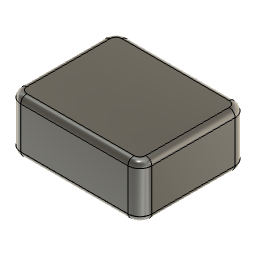
Armreif_Box v4 (Autodesk Fusion 360 design; units mm, degrees)
Autodesk Fusion 360 part; units mm, degrees
sketch "Sketch1" plane through (0, 0, 0) normal (0, 0, 1) x (1, 0, 0) in component "Base"
  line L0 (0, 0) -> (110, 0)
  line L1 (110, 0) -> (110, 90)
  line L2 (110, 90) -> (0, 90)
  line L3 (0, 90) -> (0, 0)
  dimension "d1" = 110
  dimension "d2" = 90
  constraint horizontal L0
  constraint vertical L1
  constraint horizontal L2
  constraint vertical L3
  constraint coincident L0.start L3.end
  measures "d1" distance of L0.start L0.end
  measures "d2" distance of L0.start L2.end
extrude "Extrude1" add sketch "Sketch1" along normal blind 10 makes body 1 in component "Base"
sketch "Sketch5" plane through (0, 0, 10) normal (0, 0, 1) x (-1, 0, 0) in component "Base"
  line L0 (0, -90) -> (0, 0)
  line L1 (0, 0) -> (-110, 0)
  line L2 (-110, 0) -> (-110, -90)
  line L3 (-110, -90) -> (0, -90)
  line L4 (0, -90) -> (-110, -90)
  line L5 (-110, -90) -> (-110, 0)
  line L6 (-110, 0) -> (0, 0)
  line L7 (0, 0) -> (0, -90)
  line L8 (-10, -80) -> (-100, -80)
  line L9 (-100, -80) -> (-100, -10)
  line L10 (-100, -10) -> (-10, -10)
  line L11 (-10, -10) -> (-10, -80)
  dimension "d30" = 110
  dimension "d31" = 90
  dimension "d32" = 70
  dimension "d33" = 90
  dimension "d34" = 10
  dimension "d35" = 10
  dimension "d36" = 10
  dimension "d37" = 10
  constraint horizontal L4
  constraint vertical L5
  constraint horizontal L6
  constraint vertical L7
  constraint coincident L1.end L2.start
  constraint coincident L0.start L3.end
  constraint horizontal L8
  constraint vertical L9
  constraint horizontal L10
  constraint vertical L11
  measures "d30" distance of L0.start L2.end
  measures "d31" distance of L2.end L1.end
  measures "d32" distance of L8.start L10.end
  measures "d33" distance of L8.start L8.end
  measures "d34" distance of L4 L8
  measures "d35" distance of L7 L11
  measures "d36" distance of L5 L9
  measures "d37" distance of L6 L10
extrude "Extrude5" cut sketch "Sketch5" against normal blind 5 bodies 1 in component "Base"
sketch "Sketch6" plane through (0, 0, 10) normal (0, 0, 1) x (-1, 0, 0) in component "Base"
  line L0 (-10, -80) -> (-10, -10)
  line L1 (-10, -10) -> (-100, -10)
  line L2 (-100, -10) -> (-100, -80)
  line L3 (-100, -80) -> (-10, -80)
  ellipse E0 centre (-56.2263, -44.1137) end of major axis (-86.2263, -44.1137) minor radius 22.5
  line L4 (-26.2263, -44.1137) -> (-86.2263, -44.1137) construction
  line L5 (-56.2263, -21.6137) -> (-56.2263, -66.6137) construction
  dimension "d40" = 60
  dimension "d41" = 45
  constraint coincident E0 L4.start
  constraint coincident E0 L4.end
  constraint coincident E0 L5.start
  constraint coincident E0 L5.end
  constraint horizontal L4
  measures "d40" distance of E0
extrude "Extrude6" add sketch "Sketch6" along normal blind 20 contours E0 bodies 1 in component "Base"
sketch "Sketch7" plane through (0, 0, 5) normal (0, 0, 1) x (-1, 0, 0) in component "Base"
  line L0 (-100, -10) -> (-10, -10)
  line L1 (-10, -10) -> (-10, -80)
  line L2 (-10, -80) -> (-100, -80)
  line L3 (-100, -80) -> (-100, -10)
  line L4 (0, 0) -> (-110, 0)
  line L5 (-110, 0) -> (-110, -90)
  line L6 (-110, -90) -> (0, -90)
  line L7 (0, -90) -> (0, 0)
  circle A0 centre (-5, -15) radius 2.55
  circle A1 centre (-5, -75) radius 2.55
  circle A2 centre (-105, -75) radius 2.55
  circle A3 centre (-105, -15) radius 2.55
  dimension "d45" = 5.1
  dimension "d46" = 5.1
  dimension "d47" = 5.1
  dimension "d48" = 5.1
  dimension "d49" = 5
  dimension "d50" = 5
  dimension "d51" = 5
  dimension "d52" = 5
  dimension "d53" = 60
  dimension "d54" = 60
  dimension "d55" = 15
  dimension "d56" = 15
  measures "d45" diameter of A0
  measures "d46" diameter of A1
  measures "d47" diameter of A2
  measures "d48" diameter of A3
  measures "d49" distance of L1 A1.centre
  measures "d50" distance of L1 A0.centre
  measures "d51" distance of L3 A3.centre
  measures "d52" distance of L3 A2.centre
  measures "d53" distance of A0.centre A1.centre
  measures "d54" distance of A2.centre A3.centre
  measures "d55" distance of L6 A2.centre
  measures "d56" distance of L6 A1.centre
extrude "Extrude7" cut sketch "Sketch7" against normal blind 3.1 contours A0 | A1 | A2 | A3 bodies 1 in component "Base"
sketch "Sketch1 (2)" plane through (0, 0, 0) normal (0, 0, 1) x (1, 0, 0) in component "Lid"
  line L0 (0, -45.2514) -> (110, -45.2514)
  line L1 (110, -45.2514) -> (110, -135.2514)
  line L2 (110, -135.2514) -> (0, -135.2514)
  line L3 (0, -135.2514) -> (0, -45.2514)
  dimension "d59" = 110
  dimension "d60" = 90
  constraint horizontal L0
  constraint vertical L1
  constraint horizontal L2
  constraint vertical L3
  measures "d59" distance of L0.start L0.end
  measures "d60" distance of L0.start L2.end
extrude "Extrude1'" add sketch "Sketch1 (2)" along normal blind 40 separate body makes body 2 in component "Lid"
sketch "Sketch2" plane through (0, 0, 40) normal (0, 0, 1) x (-1, 0, 0) in component "Lid"
  line L0 (0, 135.2514) -> (-110, 135.2514)
  line L1 (-110, 135.2514) -> (-110, 45.2514)
  line L2 (-110, 45.2514) -> (0, 45.2514)
  line L3 (0, 45.2514) -> (0, 135.2514)
  line L4 (-9.75, 55.0014) -> (-100.25, 55.0014)
  line L5 (-100.25, 55.0014) -> (-100.25, 125.5014)
  line L6 (-100.25, 125.5014) -> (-9.75, 125.5014)
  line L7 (-9.75, 125.5014) -> (-9.75, 55.0014)
  dimension "d63" = 90.5
  dimension "d64" = 70.5
  dimension "d65" = 9.75
  dimension "d66" = 9.75
  dimension "d67" = 9.75
  dimension "d68" = 9.75
  constraint horizontal L4
  constraint vertical L5
  constraint horizontal L6
  constraint vertical L7
  measures "d63" distance of L4.start L4.end
  measures "d64" distance of L4.start L6.end
  measures "d65" distance of L1 L5
  measures "d66" distance of L3 L7
  measures "d67" distance of L2 L4
  measures "d68" distance of L0 L6
extrude "Extrude2" cut sketch "Sketch2" against normal blind 30 contours L4 L5 L6 L7 bodies 2 in component "Lid"
fillet "Fillet1" radius 3 1 edges at (26.2263, 44.1137, 30) on bodies 1 in component "Base"
fillet "Fillet2" radius 10 8 edges at (0, 0, 2.5) (0, 90, 2.5) (110, 90, 2.5) (110, 0, 2.5) (100, 10, 7.5) (100, 80, 7.5) (10, 80, 7.5) (10, 10, 7.5) on bodies 1 in component "Base"
sketch "Sketch4" plane through (0, -45.5027, 40) normal (0, 0, 1) x (-1, 0, 0) in component "Lid"
  line L0 (-100.25, 9.4986) -> (-100.25, 79.9986)
  line L1 (-100.25, 79.9986) -> (-9.75, 79.9986)
  line L2 (-9.75, 79.9986) -> (-9.75, 9.4986)
  line L3 (-9.75, 9.4986) -> (-100.25, 9.4986)
  line L4 (0, 89.7486) -> (-110, 89.7486)
  line L5 (-110, 89.7486) -> (-110, -0.2514)
  line L6 (-110, -0.2514) -> (0, -0.2514)
  line L7 (0, -0.2514) -> (0, 89.7486)
  circle A0 centre (-105, 74.7486) radius 2.55
  circle A1 centre (-105, 14.7486) radius 2.55
  circle A2 centre (-5, 74.7486) radius 2.55
  circle A3 centre (-5, 14.7486) radius 2.55
  dimension "d89" = 5.1
  dimension "d90" = 5.1
  dimension "d91" = 5.1
  dimension "d92" = 5.1
  dimension "d93" = 5
  dimension "d94" = 5
  dimension "d95" = 5
  dimension "d96" = 5
  dimension "d97" = 60
  dimension "d98" = 60
  dimension "d99" = 15
  dimension "d100" = 15
  measures "d89" diameter of A0
  measures "d90" diameter of A1
  measures "d91" diameter of A2
  measures "d92" diameter of A3
  measures "d93" distance of L5 A0.centre
  measures "d94" distance of L5 A1.centre
  measures "d95" distance of L7 A2.centre
  measures "d96" distance of L7 A3.centre
  measures "d97" distance of A0.centre A1.centre
  measures "d98" distance of A2.centre A3.centre
  measures "d99" distance of L4 A0.centre
  measures "d100" distance of L4 A2.centre
extrude "Extrude3" cut sketch "Sketch4" against normal blind 3.1 contours A0 | A1 | A2 | A3 bodies 2 in component "Lid"
fillet "Fillet2'" radius 10 8 edges at (0, -45.2514, 20) (0, -135.2514, 20) (110, -45.2514, 20) (100.25, -125.5014, 25) (9.75, -55.0014, 25) (110, -135.2514, 20) (9.75, -125.5014, 25) (100.25, -55.0014, 25) on bodies 2 in component "Lid"
fillet "Fillet3" radius 5 8 edges at (107.0711, -48.1803, 0) (110, -90.2514, 0) (107.0711, -132.3224, 0) (55, -135.2514, 0) (2.9289, -132.3224, 0) (0, -90.2514, 0) (2.9289, -48.1803, 0) (55, -45.2514, 0) on bodies 2 in component "Lid"
fillet "Fillet3'" radius 5 8 edges at (0, 45, 0) (2.9289, 2.9289, 0) (55, 0, 0) (107.0711, 2.9289, 0) (110, 45, 0) (107.0711, 87.0711, 0) (55, 90, 0) (2.9289, 87.0711, 0) on bodies 1 in component "Base"
component "Base" placed x (1, 0, 0) y (0, 1, 0) z (0, 0, 1) at (0, 0, 0)
component "Lid" placed x (1, 0, 0) y (0, 1, 0) z (0, 0, 1) at (0, 0, 0)
